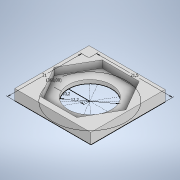
# Autodesk Inventor part: ScrewTest
Saved by Autodesk Inventor 2022 (Build 260153000, 153)
## iProperties
Created: 2022-04-20
Part Number: ScrewTest
Material: Generic
Document SubType Name: Modeling
Designer: Bruger
Density: 1 g/cm^3
Appearance: Default
Author: Bruger
Autodesk Inventor part; units mm, degrees
ref_plane "YZ Plane" through (0, 0, 0) normal (1, 0, 0) x (0, 1, 0)
ref_plane "XZ Plane" through (0, 0, 0) normal (0, 1, 0) x (-1, 0, 0)
ref_plane "XY Plane" through (0, 0, 0) normal (0, 0, 1) x (1, 0, 0)
sketch "Sketch1" plane through (0, 0, 0) normal (0, 1, 0) x (-1, 0, 0)
  line L0 (-10.75, 10.5) -> (10.75, 10.5)
  line L1 (10.75, 10.5) -> (10.75, -10.5)
  line L2 (10.75, -10.5) -> (-10.75, -10.5)
  line L3 (-10.75, -10.5) -> (-10.75, 10.5)
  line L4 (-10.75, 10.5) -> (10.75, -10.5) construction
  line L5 (10.75, 10.5) -> (-10.75, -10.5) construction
  circle A0 centre (0, 0) radius 6.1
  line L6 (0, 0) -> (9, 0) construction
  line L7 (0, 0) -> (9, 0) construction
  line L8 (0, 0) -> (10.2, 0) construction
  line L9 (0, 0) -> (9, 0) construction
  line L10 (0, 0) -> (10.2, 0)
  line L11 (0, 0) -> (5.1, 8.8335) construction
  line L12 (0, 0) -> (-5.1, 8.8335) construction
  line L13 (0, 0) -> (-10.2, 0) construction
  line L14 (0, 0) -> (-5.1, -8.8335) construction
  line L15 (0, 0) -> (5.1, -8.8335) construction
  line L16 (10.35, -0.2598) -> (5.4, -8.8335)
  line L17 (5.4, -8.8335) -> (-5.1, -8.8335)
  line L18 (-5.1, -8.8335) -> (-10.2, 0)
  line L19 (-10.2, 0) -> (-5.1, 8.8335)
  line L20 (-5.1, 8.8335) -> (5.1, 8.8335)
  line L21 (5.1, 8.8335) -> (10.35, -0.2598)
  dimension "d0" = 21.5
  dimension "d1" = 21
  dimension "d2" = 12.2
  dimension "d28" = 10.2
  dimension "d31" = 360
  constraints: 44 end point, 7 horizontal, 5 parallel, 2 midpoint, 1 centre point, 1 coincident, 1 perpendicular, 19 other
  measures "d0" distance of L1.end L2.end
  measures "d1" distance of L0.end L1.end
  measures "d2" diameter of A0
  measures "d28" distance of L10.start L8.end
extrude "Extrusion1" add sketch "Sketch1" along normal blind 3 contours L0 L1 L2 L3 | A0 | L21 L16 L17 L18 L19 L20
extrude "Extrusion6" cut sketch "Sketch1" along normal blind 12.2 contours A0 | L21 L16 L17 L18 L19 L20
extrude "Extrusion7" add sketch "Sketch1" along normal blind 1 contours L21 L16 L17 L18 L19 L20
equation "\"d33\" = d2"
body "Solid1"
